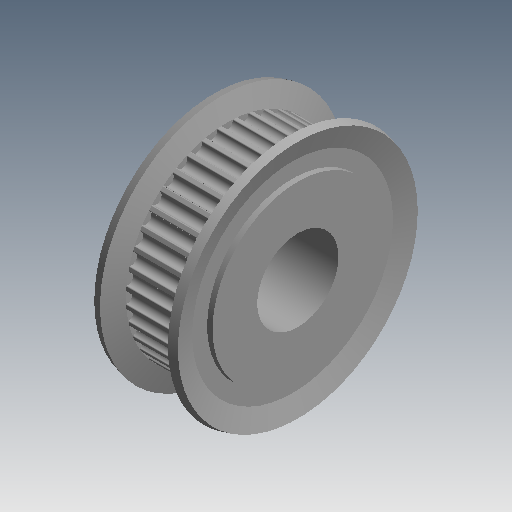
# Autodesk Inventor part: GPA40GT2060-A-H10_b
Saved by Autodesk Inventor 2020.1 (Build 241239000, 239)
## iProperties
Part Number: GPA40GT2060-A-H10_b
Material: 一般
Catalog Web Link: www.cadenas.de
Description: GPA__GT2040, GPA__GT2060, GPA__GT2090_body-High Torque Timing Pulleys 2GT Type
Vendor: MISUMI
Document SubType Name: Modeling
Designer: partserver
Manufacturer: MISUMI
Mass: 4.24044 g
Surface Area: 31.018 cm^2
Volume: 4.24044 cm^3
Density: 1 g/cm^3
Appearance: PSOLRGB-192-192-192
Category: PARTsolutions
Company: MISUMI
PSOL_IDENT_0: {$CADENAS_DATA\23d-libs\misumi\metric\51_timing_pulleys\gpa__gt2\gpa_gt2.prj},385 {VTYP=3D},{NB=GPA4
PSOL_IDENT_1: 0GT2060-A-H10_b},{LINA=GPA40GT2060-A-H10},{NN=GPA__GT2040, GPA__GT2060, GPA__GT2090_body},{DATE=17.0
PSOL_IDENT_2: 1.2019 09:47:54},{GEOMDATE=17.12.2018 08:21:00},{VERSION=},{LINEID=250},{WBVAR=TNW,PS,SBS,DD,Z,J,Q,R
PSOL_IDENT_3: ,S,T,ALT1,ALT2,M,QSC,QFC,QTC,ALT3,K,KSC,KFC,KTC,ALT4,ZM,ZSC,ZFC,ZTC,ALT5,BC,ALT6,ALT7,ALT8,FC},{WBNU
PSOL_IDENT_4: MERIC=DD,Z,J,Q,R,S,T,QSC,QFC,QTC,K,KSC,KFC,KTC,ZSC,ZFC,ZTC,BC,FC}  {NB=GPA40GT2060-A-H10_b},{LINA=GP
PSOL_IDENT_5: A40GT2060-A-H10},{KT=DUMMY},{PN=GPA40GT2060-A-H10},{TYPE=GPA},{NT=40},{TNW=GT2060},{BW=6},{A=7.0},{W=
PSOL_IDENT_6: 10.3},{L=18.0},{PS=A},{PSA= 'A','B' },{SBS=H},{SBSALG= 'H','Round Hole','P','Round Hole+Tap','N','Ne
PSOL_IDENT_7: w JIS Keywayed Bore + Tap (Standard)','NK','New JIS Keywayed Bore + Tap (keyway width 4.0mm, height
PSOL_IDENT_8: 1.8mm)','V','Stepped Hole','Y','Both Ends Stepped Hole' },{DD=10.00},{DDALG=[6:6/1],[6.35],[7:17/1]}
PSOL_IDENT_9: ,{DDHA=[6:6/1],[6.35],[7:17/1]},{DDHB=[6:6/1],[6.35],[7:13/1]},{DDPA=[6:6/1],[6.35],[7:12/1]},{DDPB=
PSOL_IDENT_10: [6:6/1],[6.35],[7:10/1]},{DDNA=8,10},{DDNB=},{DDNKA=[10:10/1]},{DDNKB=0},{DDVA=[6:6/1],[6.35],[7:15/
PSOL_IDENT_11: 1]},{DDVFB=[6:6/1],[6.35],[7:11/1]},{DDYA=[6:15/1]},{Z=0},{ZALG=0},{ZMIN=12},{ZAMAX=17},{ZBMAX=13},{
PSOL_IDENT_12: J=0.0},{JALG=0},{JMAX=8.3},{Q=0},{R=0},{QRALG=0},{QRMIN=12},{QRMAX=17},{S=0.0},{SALG=0},{SMAX=4.300}
PSOL_IDENT_13: ,{T=0.0},{TALG=0},{TMAX=5.000},{PD=25.46},{OD=24.95},{D=17},{DE=21},{DDZ=10},{F=30},{E=21},{BB=0},{T
PSOL_IDENT_14: T=0},{M1=4},{AC=-},{ALT1=},{ALT1A= '','Not applicable' },{ANG=117},{ALT2=},{ALT2A= '','Not applicabl
PSOL_IDENT_15: e' },{M=N/A},{MALG= 'N/A' },{MM=0.000},{MPHD=0.000},{MA= 'N/A' },{MSA= 'N/A' },{QSC=0.0},{QSCA=0},{Q
PSOL_IDENT_16: FC=0.0},{QFCA=0},{QTC=0.0},{QTCA=0},{QPCDMIN=14},{QPCDMINALG=14},{QPCDMAX=17},{ALT2PN=},{ALT3=},{ALT
PSOL_IDENT_17: 3A= '','Not applicable' },{K=0.0},{KA=0},{KAMIN=4},{KAMAX=0},{KSMAX=0},{KSC=0.0},{KSCA=0},{KFC=0.0},
PSOL_IDENT_18: {KFCA=0},{KTC=0.0},{KTCA=0},{KSCMIN=14.000},{KPCDMIN=14.000},{KPCDMINALG=18.000},{KPCDMAX=17.000},{A
PSOL_IDENT_19: LT3PN=},{ALT4=},{ALT4ALG= '','Not applicable' },{ALT4MIN=20.500},{ALT4MAX=10.500},{ZM=N/A},{ZMALG= '
PSOL_IDENT_20: N/A' },{ZMFTALG= 'N/A' },{ZMSALG= 'N/A' },{ZMDD1=0.0},{ZMDD2=0.0},{ZMHH=0.0},{ZSC=0.0},{ZSCALG=[0]},
PSOL_IDENT_21: {ZFC=0.0},{ZFCALG=[0]},{ZTC=0.0},{ZTCALG=[0]},{ZPCDMIN=0.000},{ZPCDMINALG=0.000},{ZPCDMAX=17.000},{A
PSOL_IDENT_22: LT4PN=},{ALT5=},{ALT5ALG= '','Not applicable' },{ALT5PN=},{BC=0.0},{BCALG=0},{BCMIN=3.000},{BCMAX=7.
PSOL_IDENT_23: 700},{ALT6=},{ALT7=},{ALT7ALG= '','w/o Flange Attached on One Side Only','-RFC','with RFC (Flange At
PSOL_IDENT_24: tached on The Boss Side Only)','-LFC','with LFC (Flange Attached on The Opposite Side Only)' },{ALT8=
PSOL_IDENT_25: },{ALT8ALG='','w/o FC (Flange Cut)','-FC','with FC (Flange Cut)'},{ALT8PN=},{FC=0.0},{FCA=0},{ODAINT=
PSOL_IDENT_26: 28.000},{FCMIN=26},{FCMAX=28},{WLBC=10.3},{SL=5},{SL2=5},{KTT=5},{KYY=7.475},{TAP=0}
NB: GPA40GT2060-A-H10_b
NN: GPA__GT2040, GPA__GT2060, GPA__GT2090_body
NT: 40
NBSYN: $PN._b
LINA: GPA40GT2060-A-H10
CATALOG: Misumi
PN: GPA40GT2060-A-H10
TNW: GT2060
A: 7
W: 10.3
L: 18
PS: A
SBS: Round Hole
DD: 10
Z: 0
J: 0
Q: 0
R: 0
S: 0
T: 0
PD: 25.46
OD: 24.95
D: 17
F: 30
E: 21
AC: -
ALT1: Not applicable
ALT2: Not applicable
M: N/A
QSC: 0
QFC: 0
QTC: 0
ALT3: Not applicable
K: 0
KSC: 0
KFC: 0
KTC: 0
ALT4: Not applicable
ZM: N/A
ZMDD1: 0
ZMDD2: 0
ZMHH: 0
ZSC: 0
ZFC: 0
ZTC: 0
ALT5: Not applicable
BC: 0
ALT6: w/o Flange not Attached
ALT7: w/o Flange Attached on One Side Only
ALT8: w/o FC (Flange Cut)
FC: 0
SUPPLIER: MISUMI
ARTICLENO: GPA40GT2060-A-H10_b
BOMINFO: GPA40GT2060-A-H10
CREATOR: CADENAS GmbH
Title: GPA40GT2060-A-H10
Author: Cadenas PARTsolutions
Comments: High Torque Timing Pulleys 2GT Type
Autodesk Inventor part; units mm, degrees
ref_plane "YZ Plane" through (0, 0, 0) normal (1, 0, 0) x (0, 1, 0)
ref_plane "XZ Plane" through (0, 0, 0) normal (0, 1, 0) x (-1, 0, 0)
ref_plane "XY Plane" through (0, 0, 0) normal (0, 0, 1) x (1, 0, 0)
sketch "Sketch_16" plane through (0, 0, 0) normal (0, 0, 1) x (1, 0, 0)
  line L0 (5.15, 0) -> (-5.15, 0)
  line L1 (-5.15, 0) -> (-5.15, 10.5)
  line L2 (-5.15, 10.5) -> (-3.5, 10.5)
  line L3 (-3.5, 10.5) -> (-3.5, 12.475)
  line L4 (-3.5, 12.475) -> (3.5, 12.475)
  line L5 (3.5, 12.475) -> (3.5, 10.5)
  line L6 (3.5, 10.5) -> (5.15, 10.5)
  line L7 (5.15, 10.5) -> (5.15, 0)
  line L8 (5.15, 0) -> (-5.15, 0)
  constraints: 18 end point
revolve "Revolution1" add sketch "Sketch_16" angle 360 about axis through (5.15, 0, 0) along (1, 0, 0)
sketch "Sketch_18" plane through (0, 0, 0) normal (1, 0, 0) x (0, 1, 0)
  line L0 (12.6944, 0.9513) -> (12.4419, 0.9324)
  line L1 (12.4419, 0.9324) -> (12.4509, 0.7917)
  arc A0 (12.3479, 0.6729) -> (12.4509, 0.7917) centre (12.3391, 0.7846) ccw
  arc A1 (12.3479, 0.6729) -> (12.3479, -0.6729) centre (12.401, 0) ccw
  arc A2 (12.4509, -0.7917) -> (12.3479, -0.6729) centre (12.3391, -0.7846) ccw
  line L2 (12.4509, -0.7917) -> (12.4419, -0.9324)
  line L3 (12.4419, -0.9324) -> (12.6944, -0.9513)
  arc A3 (12.6944, -0.9513) -> (12.6944, 0.9513) centre (0, 0) ccw
  constraints: 8 end point, 8 point on circle, 4 centre point
extrude "Extrusion1" cut sketch "Sketch_18" along normal mid plane 7
pattern_circular "Circular Pattern1" count 40 over 360 about axis through (0, 0, 0) along (1, 0, 0) of "Extrusion1"
sketch "Sketch_20" plane through (0, 0, 0) normal (0, 0, 1) x (1, 0, 0)
  line L0 (50, 0) -> (-50, 0)
  line L1 (3.5, 12.475) -> (3.5, 10.5)
  line L2 (3.5, 10.5) -> (4.5, 10.5)
  line L3 (4.5, 10.5) -> (4.5, 12.3433)
  line L4 (4.5, 12.3433) -> (5.1425, 14.7412)
  line L5 (5.1425, 14.7412) -> (4.1766, 15)
  line L6 (4.1766, 15) -> (3.5, 12.475)
  constraints: 14 end point
revolve "Revolution2" add sketch "Sketch_20" angle 360 about axis through (50, 0, 0) along (1, 0, 0)
sketch "Sketch_21" plane through (0, 0, 0) normal (0, 0, 1) x (1, 0, 0)
  line L0 (50, 0) -> (-50, 0)
  line L1 (-5.1425, 14.7412) -> (-4.5, 12.3433)
  line L2 (-4.5, 12.3433) -> (-4.5, 10.5)
  line L3 (-4.5, 10.5) -> (-3.5, 10.5)
  line L4 (-3.5, 10.5) -> (-3.5, 12.475)
  line L5 (-3.5, 12.475) -> (-4.1766, 15)
  line L6 (-4.1766, 15) -> (-5.1425, 14.7412)
  constraints: 14 end point
revolve "Revolution3" add sketch "Sketch_21" angle 360 about axis through (50, 0, 0) along (1, 0, 0)
sketch "Sketch5" plane through (5.15, 0, 0) normal (1, 0, 0) x (0, 0, -1)
  point P0 (0, 0)
hole "Hole1" at (5.15, 0, 0) direction (-1, 0, 0) diameter 10 depth 10.3
body "Solid1"
